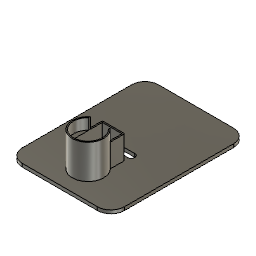
7ad9df1d-be35-4644-bc9c-72c505da536f (Autodesk Fusion 360 design; units mm, degrees)
part number: 2026-05-17-07-30-09-330
Autodesk Fusion 360 part; units mm, degrees
note: some values were not read from the file. Set by a fixed rule: which sketch regions a step uses.
sketch "スケッチ1" plane through (0, 0, 0) normal (0, 0, 1) x (1, 0, 0)
  line L0 (20, 0) -> (130, 0)
  line L1 (150, 20) -> (150, 180)
  line L2 (130, 200) -> (20, 200)
  line L3 (0, 180) -> (0, 20)
  arc A0 (20, 200) -> (0, 180) centre (20, 180) ccw
  arc A1 (150, 180) -> (130, 200) centre (130, 180) ccw
  arc A2 (0, 20) -> (20, 0) centre (20, 20) ccw
  arc A3 (130, 0) -> (150, 20) centre (130, 20) ccw
  point P0 (150, 0)
  point P1 (0, 200)
  dimension "d1" = 150
  dimension "d2" = 200
  dimension "d5" = 20
  dimension "d6" = 20
  dimension "d7" = 20
  dimension "d8" = 20
  constraint horizontal L0
  constraint vertical L1
  constraint horizontal L2
  constraint vertical L3
  constraint coincident P1 L2
  constraint coincident P1 L3
  constraint tangent L2 A0
  constraint tangent L3 A0
  constraint tangent L1 A1
  constraint tangent L2 A1
  constraint coincident origin L0
  constraint coincident origin L3
  constraint tangent L0 A2
  constraint tangent L3 A2
  constraint coincident P0 L0
  constraint coincident P0 L1
  constraint tangent L0 A3
  constraint tangent L1 A3
  measures "d1" distance of origin P0
  measures "d2" distance of origin P1
  measures "d5" radius of A0
  measures "d6" radius of A1
  measures "d7" radius of A2
  measures "d8" radius of A3
extrude "押し出し1" add sketch "スケッチ1" along normal blind 5
sketch "スケッチ2" plane through (0, 0, 5) normal (0, 0, 1) x (-1, 0, 0)
  arc A0 (-130, 0) -> (-150, -20) centre (-130, -20) ccw
  arc A1 (-150, -180) -> (-130, -200) centre (-130, -180) ccw
  line L0 (-130, -200) -> (-20, -200)
  arc A2 (-20, -200) -> (0, -180) centre (-20, -180) ccw
  arc A3 (0, -20) -> (-20, 0) centre (-20, -20) ccw
  line L1 (-20, 0) -> (-130, 0)
  line L2 (-89.4, -30) -> (-60.6, -30)
  line L3 (-60.6, -30) -> (-60.6, -76.8)
  line L4 (-60.6, -76.8) -> (-89.4, -76.8)
  line L5 (-89.4, -76.8) -> (-89.4, -30)
  line L6 (-91.4, -28) -> (-58.6, -28)
  line L7 (-58.6, -28) -> (-58.6, -78.8)
  line L8 (-58.6, -78.8) -> (-91.4, -78.8)
  line L9 (-91.4, -78.8) -> (-91.4, -28)
  line L10 (0, -180) -> (0, -20)
  dimension "d9" = 28.8
  dimension "d10" = 46.8
  dimension "d11" = 150
  dimension "d12" = 200
  dimension "d13" = 60.6
  dimension "d14" = 30
  dimension "d15" = 32.8
  dimension "d16" = 50.8
  dimension "d17" = 58.6
  dimension "d18" = 28
  constraint horizontal L2
  constraint vertical L3
  constraint horizontal L4
  constraint vertical L5
  constraint horizontal L6
  constraint vertical L7
  constraint horizontal L8
  constraint vertical L9
  measures "d9" distance of L2.start L2.end
  measures "d10" distance of L2.end L3.end
  measures "d11" distance of A1.start L10
  measures "d12" distance of L0 L1
  measures "d13" distance of A0.end L5
  measures "d14" distance of L1 L2
  measures "d15" distance of L7 L9
  measures "d16" distance of L6 L8
  measures "d17" distance of A0.end L9
  measures "d18" distance of L1 L6
extrude "押し出し2" add sketch "スケッチ2" along normal blind 34
sketch "スケッチ3" plane through (0, 0, 39) normal (0, 0, 1) x (-1, 0, 0)
  line L0 (-60.6, -76.8) -> (-89.4, -76.8)
  line L1 (-89.4, -76.8) -> (-89.4, -30)
  line L2 (-89.4, -30) -> (-60.6, -30)
  line L3 (-60.6, -30) -> (-60.6, -76.8)
  line L4 (-91.4, -78.8) -> (-58.6, -78.8)
  line L5 (-58.6, -78.8) -> (-58.6, -28)
  line L6 (-58.6, -28) -> (-91.4, -28)
  line L7 (-91.4, -28) -> (-91.4, -78.8)
  circle A0 centre (-75, -41.3) radius 21.25
  circle A1 centre (-75, -41.3) radius 23
  dimension "d21" = 42.5
  dimension "d22" = 11.3
  dimension "d23" = 46
  constraint concentric A0 A1
  measures "d21" diameter of A0
  measures "d22" distance of L2 A0.centre
  measures "d23" diameter of A1
extrude "押し出し3" add sketch "スケッチ3" against normal blind 2 contours L5 L6 L7 A0
extrude "押し出し4" add sketch "スケッチ3" along normal blind 16 and the other way blind 34 contours L3 L5 A0 A1 | L1 L7 A0 A1 | L5 L7 A0 A1
fillet "フィレット1" radius 1 1 edges at (91.4, 78.8, 22)
fillet "フィレット2" radius 1 1 edges at (58.6, 78.8, 22)
sketch "スケッチ4" plane through (0, 0, 5) normal (0, 0, 1) x (-1, 0, 0)
  line L0 (-60.6, -76.8) -> (-60.6, -30)
  line L1 (-60.6, -30) -> (-89.4, -30)
  line L2 (-89.4, -30) -> (-89.4, -76.8)
  line L3 (-89.4, -76.8) -> (-60.6, -76.8)
  line L4 (-89.4, -46) -> (-60.6, -46)
  line L5 (-60.6, -46) -> (-60.6, -66)
  line L6 (-60.6, -66) -> (-89.4, -66)
  line L7 (-89.4, -66) -> (-89.4, -46)
  dimension "d35" = 16
  dimension "d36" = 20
  constraint horizontal L4
  constraint vertical L5
  constraint horizontal L6
  constraint vertical L7
  constraint coincident L0 L5.end
  constraint coincident L2 L4.start
  measures "d35" distance of L1 L4
  measures "d36" distance of L4 L6
extrude "押し出し5" cut sketch "スケッチ4" against normal up to surface (5 mm away) contours L0 L2 L4 L5 L6 L7
sketch "スケッチ5" plane through (0, 0, 0) normal (0, 0, -1) x (1, 0, 0)
  line L0 (89.4, -46) -> (89.4, -66)
  line L1 (89.4, -66) -> (60.6, -66)
  line L2 (60.6, -66) -> (60.6, -46)
  line L3 (60.6, -46) -> (89.4, -46)
  arc A0 (150, -20) -> (130, 0) centre (130, -20) ccw
  line L4 (130, 0) -> (20, 0)
  arc A1 (20, 0) -> (0, -20) centre (20, -20) ccw
  line L5 (0, -20) -> (0, -180)
  arc A2 (0, -180) -> (20, -200) centre (20, -180) ccw
  line L6 (20, -200) -> (130, -200)
  arc A3 (130, -200) -> (150, -180) centre (130, -180) ccw
  line L7 (150, -180) -> (150, -20)
  circle A4 centre (64, -33.4) radius 2.6
  circle A5 centre (86, -73.4) radius 2.6
  circle A6 centre (86, -33.4) radius 2.6
  circle A7 centre (64, -73.4) radius 2.6
  line L8 (75, -25) -> (75, -85)
  line L9 (89.4, -30) -> (60.6, -30)
  line L10 (60.6, -76.8) -> (89.4, -76.8)
  circle A8 centre (64, -33.4) radius 1.4
  circle A9 centre (86, -33.4) radius 1.4
  circle A10 centre (64, -73.4) radius 1.4
  circle A11 centre (86, -73.4) radius 1.4
  dimension "d39" = 5.2
  dimension "d40" = 5.2
  dimension "d41" = 5.2
  dimension "d42" = 5.2
  dimension "d43" = 22
  dimension "d44" = 22
  dimension "d45" = 40
  dimension "d46" = 40
  dimension "d47" = 75
  dimension "d48" = 11
  dimension "d49" = 11
  dimension "d50" = 46.8
  dimension "d51" = 3.4
  dimension "d52" = 3.4
  dimension "d53" = 2.8
  dimension "d54" = 2.8
  dimension "d55" = 2.8
  dimension "d56" = 2.8
  constraint perpendicular L1 L8
  constraint concentric A4 A8
  constraint concentric A6 A9
  constraint concentric A7 A10
  constraint concentric A5 A11
  measures "d39" diameter of A4
  measures "d40" diameter of A5
  measures "d41" diameter of A6
  measures "d42" diameter of A7
  measures "d43" distance of A4.centre A6.centre
  measures "d44" horizontal distance of A5.centre A7.centre
  measures "d45" vertical distance of A5.centre A6.centre
  measures "d46" vertical distance of A4.centre A7.centre
  measures "d47" distance of L5 L8
  measures "d48" distance of A4.centre L8
  measures "d49" distance of A7.centre L8
  measures "d50" distance of L9 L10
  measures "d51" distance of A6.centre L9
  measures "d52" distance of A4.centre L9
  measures "d53" diameter of A8
  measures "d54" diameter of A9
  measures "d55" diameter of A10
  measures "d56" diameter of A11
extrude "押し出し6" cut sketch "スケッチ5" against normal blind 5 contours A8 | A9 | A10 | A11
extrude "押し出し7" cut sketch "スケッチ5" against normal blind 4 contours A4 | A5 | A6 | A7
sketch "スケッチ6" plane through (0, 0, 5) normal (0, 0, 1) x (-1, 0, 0)
  arc A0 (-58.6, -57.4258) -> (-91.4, -57.4258) centre (-75, -41.3) ccw
  line L0 (-58.6, -57.4258) -> (-58.6, -77.8)
  arc A1 (-59.6, -78.8) -> (-58.6, -77.8) centre (-59.6, -77.8) ccw
  line L1 (-59.6, -78.8) -> (-90.4, -78.8)
  arc A2 (-91.4, -77.8) -> (-90.4, -78.8) centre (-90.4, -77.8) ccw
  line L2 (-91.4, -77.8) -> (-91.4, -57.4258)
  arc A3 (-130, 0) -> (-150, -20) centre (-130, -20) ccw
  line L3 (-150, -20) -> (-150, -180)
  arc A4 (-150, -180) -> (-130, -200) centre (-130, -180) ccw
  line L4 (-130, -200) -> (-20, -200)
  arc A5 (-20, -200) -> (0, -180) centre (-20, -180) ccw
  line L5 (0, -180) -> (0, -20)
  arc A6 (0, -20) -> (-20, 0) centre (-20, -20) ccw
  line L6 (-20, 0) -> (-130, 0)
  circle A7 centre (-90, -90) radius 5
  circle A8 centre (-60, -90) radius 5
  line L7 (-90, -85) -> (-60, -85)
  line L8 (-60, -85) -> (-60, -95)
  line L9 (-60, -95) -> (-90, -95)
  line L10 (-90, -95) -> (-90, -85)
  dimension "d61" = 10
  dimension "d62" = 10
  constraint horizontal L7
  constraint vertical L8
  constraint horizontal L9
  constraint vertical L10
  constraint coincident A8 L8.end
  constraint coincident A7 L7.start
  measures "d61" diameter of A7
  measures "d62" diameter of A8
extrude "押し出し8" cut sketch "スケッチ6" against normal blind 5 contours A7 L10 | A7 A8 L7 L9 | A7 L10 | A8 L8 | A8 L8
equation "d13 = ( 150 mm - d9 ) / 2"
equation "d15 = d9 + 4 mm"
equation "d16 = d10 + 4 mm"
equation "d17 = ( d11 - d15 ) / 2"
equation "d18 = d14 - 2 mm"
equation "d44 = d43"
equation "d46 = d45"
equation "d48 = d43 / 2"
equation "d49 = d48"
equation "d51 = ( d50 - d45 ) / 2"
equation "d52 = d51"
